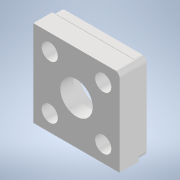
# Autodesk Inventor part: Part8
Saved by Autodesk Inventor 2020.2 (Build 242310000, 310)
## iProperties
Created: 2022-11-14
Part Number: Part8
Material: 一般
Document SubType Name: Modeling
Designer: Administrator
Density: 1 g/cm^3
Appearance: 既定
Author: Administrator
Autodesk Inventor part; units mm, degrees
ref_plane "YZ Plane" through (0, 0, 0) normal (1, 0, 0) x (0, 1, 0)
ref_plane "XZ Plane" through (0, 0, 0) normal (0, 1, 0) x (-1, 0, 0)
ref_plane "XY Plane" through (0, 0, 0) normal (0, 0, 1) x (1, 0, 0)
sketch "スケッチ1" plane through (0, 0, 0) normal (0, 0, 1) x (1, 0, 0)
  circle A0 centre (0.0113, -0.6482) radius 9.5 projected
  circle A1 centre (0.0113, -0.6482) radius 5 projected
  circle A2 centre (0.0113, -0.6482) radius 5 projected
  circle A3 centre (0.0113, -0.6482) radius 14
  circle A4 centre (-9.8882, 9.2513) radius 1.5
  circle A5 centre (9.9108, -10.5477) radius 1.5
  line L0 (0.0113, -0.6482) -> (9.9108, 9.2513)
  line L1 (0.0113, -0.6482) -> (14.0113, -0.6482) construction
  line L2 (0.0113, -0.6482) -> (-9.8882, 9.2513)
  line L3 (0.0113, -0.6482) -> (14.0113, -0.6482) construction
  line L4 (0.0113, -0.6482) -> (-9.8882, -10.5477)
  line L5 (0.0113, -0.6482) -> (14.0113, -0.6482) construction
  line L6 (0.0113, -0.6482) -> (9.9108, -10.5477)
  line L7 (0.0113, -0.6482) -> (14.0113, -0.6482) construction
  circle A6 centre (9.9108, 9.2513) radius 1.5
  circle A7 centre (-9.8882, -10.5477) radius 1.5
  circle A8 centre (-9.8882, 9.2513) radius 3
  circle A9 centre (9.9108, 9.2513) radius 3
  circle A10 centre (9.9108, -10.5477) radius 3
  circle A11 centre (-9.8882, -10.5477) radius 3
  circle A12 centre (0.0113, -0.6482) radius 6
  line L8 (-15.9887, 15.3518) -> (16.0113, 15.3518)
  line L9 (16.0113, 15.3518) -> (16.0113, -16.6482)
  line L10 (16.0113, -16.6482) -> (-15.9887, -16.6482)
  line L11 (-15.9887, -16.6482) -> (-15.9887, 15.3518)
  line L12 (-15.9887, 15.3518) -> (16.0113, -16.6482) construction
  line L13 (16.0113, 15.3518) -> (-15.9887, -16.6482) construction
  point P0 (0, 0)
  dimension "d0" = 28
  dimension "d1" = 3
  dimension "d2" = 3
  dimension "d3" = 45
  dimension "d4" = 135
  dimension "d5" = 135
  dimension "d6" = 45
  dimension "d7" = 3
  dimension "d8" = 3
  dimension "d9" = 6
  dimension "d10" = 6
  dimension "d11" = 6
  dimension "d12" = 6
  dimension "d13" = 12
  dimension "d14" = 32
  dimension "d15" = 32
  constraints: 28 end point, 10 centre point, 8 coincident, 5 horizontal, 4 equal length, 4 point on circle, 2 midpoint, 2 parallel, 1 perpendicular
  measures "d0" diameter of A3
  measures "d1" diameter of A4
  measures "d2" diameter of A5
  measures "d3" angle of L1 L0
  measures "d4" angle of L3 L2
  measures "d5" angle of L4 L5
  measures "d6" angle of L6 L7
  measures "d7" diameter of A6
  measures "d8" diameter of A7
  measures "d9" diameter of A8
  measures "d10" diameter of A9
  measures "d11" diameter of A10
  measures "d12" diameter of A11
  measures "d13" diameter of A12
  measures "d14" distance of L9.end L10.end
  measures "d15" distance of L8.end L9.end
extrude "押し出し1" add sketch "スケッチ1" along normal blind 3 contours A0 L0 A9 A3 A10 L6 | A0 L2 A8 A3 A9 L0 | L6 A10 A3 A11 L4 A0 | A0 L4 A11 A3 A8 L2 | A9 A3 A6 L0 | L0 A6 A3 A9 | A10 A3 A5 L6 | L6 A5 A3 A10 | A8 A3 A4 L2 | L2 A4 A3 A8 | A9 A3 A6 | A11 A3 A7 L4 | L4 A7 A3 A11 | A10 A3 A5 | A8 A3 A4 | A3 A7 A11 | L8 L9 L10 L11
sketch "スケッチ2" plane through (0, 0, 3) normal (0, 0, 1) x (1, 0, 0)
  circle A0 centre (0, -0.75) radius 9.5
  circle A1 centre (0, -0.75) radius 5
  circle A2 centre (0, -0.75) radius 5
  circle A3 centre (0, -0.75) radius 14
  circle A4 centre (-9.8995, 9.1495) radius 1.5
  circle A5 centre (9.8995, -10.6495) radius 1.5
  line L0 (0, -0.75) -> (9.8995, 9.1495)
  line L1 (0, -0.75) -> (14, -0.75) construction
  line L2 (0, -0.75) -> (-9.8995, 9.1495)
  line L3 (0, -0.75) -> (14, -0.75) construction
  line L4 (0, -0.75) -> (-9.8995, -10.6495)
  line L5 (0, -0.75) -> (14, -0.75) construction
  line L6 (0, -0.75) -> (9.8995, -10.6495)
  line L7 (0, -0.75) -> (14, -0.75) construction
  circle A6 centre (9.8995, 9.1495) radius 1.5
  circle A7 centre (-9.8995, -10.6495) radius 1.5
  circle A8 centre (-9.8995, 9.1495) radius 3
  circle A9 centre (9.8995, 9.1495) radius 3
  circle A10 centre (9.8995, -10.6495) radius 3
  circle A11 centre (-9.8995, -10.6495) radius 3
  circle A12 centre (0, -0.75) radius 6
  line L8 (-16, 15.25) -> (16, 15.25)
  line L9 (16, 15.25) -> (16, -16.75)
  line L10 (16, -16.75) -> (-16, -16.75)
  line L11 (-16, -16.75) -> (-16, 15.25)
  line L12 (-16, 15.25) -> (16, -16.75) construction
  line L13 (16, 15.25) -> (-16, -16.75) construction
  point P0 (0, 0)
  point P1 (0, 0)
  dimension "d18" = 28
  dimension "d19" = 3
  dimension "d20" = 3
  dimension "d21" = 45
  dimension "d22" = 135
  dimension "d23" = 135
  dimension "d24" = 45
  dimension "d25" = 3
  dimension "d26" = 3
  dimension "d27" = 6
  dimension "d28" = 6
  dimension "d29" = 6
  dimension "d30" = 6
  dimension "d31" = 12
  dimension "d32" = 32
  dimension "d33" = 32
  constraints: 28 end point, 13 centre point, 8 coincident, 5 horizontal, 4 equal length, 4 point on circle, 2 midpoint, 2 parallel, 1 perpendicular
  measures "d18" diameter of A3
  measures "d19" diameter of A4
  measures "d20" diameter of A5
  measures "d21" angle of L1 L0
  measures "d22" angle of L3 L2
  measures "d23" angle of L4 L5
  measures "d24" angle of L6 L7
  measures "d25" diameter of A6
  measures "d26" diameter of A7
  measures "d27" diameter of A8
  measures "d28" diameter of A9
  measures "d29" diameter of A10
  measures "d30" diameter of A11
  measures "d31" diameter of A12
  measures "d32" distance of L9.end L10.end
  measures "d33" distance of L8.end L9.end
extrude "押し出し2" add sketch "スケッチ2" along normal blind 2 contours A0 L0 A9 A3 A10 L6 | A0 L2 A8 A3 A9 L0 | L6 A10 A3 A11 L4 A0 | A0 L4 A11 A3 A8 L2 | L8 L9 L10 L11
sketch "スケッチ3" plane through (0, 0, 5) normal (0, 0, 1) x (1, 0, 0)
  circle A0 centre (0, -0.75) radius 9.5
  circle A1 centre (0, -0.75) radius 5
  circle A2 centre (0, -0.75) radius 5
  circle A3 centre (0, -0.75) radius 14
  circle A4 centre (-9.8995, 9.1495) radius 1.5
  circle A5 centre (9.8995, -10.6495) radius 1.5
  line L0 (0, -0.75) -> (9.8995, 9.1495)
  line L1 (0, -0.75) -> (14, -0.75) construction
  line L2 (0, -0.75) -> (-9.8995, 9.1495)
  line L3 (0, -0.75) -> (14, -0.75) construction
  line L4 (0, -0.75) -> (-9.8995, -10.6495)
  line L5 (0, -0.75) -> (14, -0.75) construction
  line L6 (0, -0.75) -> (9.8995, -10.6495)
  line L7 (0, -0.75) -> (14, -0.75) construction
  circle A6 centre (9.8995, 9.1495) radius 1.5
  circle A7 centre (-9.8995, -10.6495) radius 1.5
  circle A8 centre (-9.8995, 9.1495) radius 3
  circle A9 centre (9.8995, 9.1495) radius 3
  circle A10 centre (9.8995, -10.6495) radius 3
  circle A11 centre (-9.8995, -10.6495) radius 3
  circle A12 centre (0, -0.75) radius 6
  line L8 (-16, 15.25) -> (16, 15.25)
  line L9 (16, 15.25) -> (16, -16.75)
  line L10 (16, -16.75) -> (-16, -16.75)
  line L11 (-16, -16.75) -> (-16, 15.25)
  line L12 (-16, 15.25) -> (16, -16.75) construction
  line L13 (16, 15.25) -> (-16, -16.75) construction
  point P0 (0, 0)
  point P1 (0, 0)
  point P2 (0, 0)
  dimension "d36" = 28
  dimension "d37" = 3
  dimension "d38" = 3
  dimension "d39" = 45
  dimension "d40" = 135
  dimension "d41" = 135
  dimension "d42" = 45
  dimension "d43" = 3
  dimension "d44" = 3
  dimension "d45" = 6
  dimension "d46" = 6
  dimension "d47" = 6
  dimension "d48" = 6
  dimension "d49" = 12
  dimension "d50" = 32
  dimension "d51" = 32
  constraints: 28 end point, 13 centre point, 8 coincident, 5 horizontal, 4 equal length, 4 point on circle, 2 midpoint, 2 parallel, 1 perpendicular
  measures "d36" diameter of A3
  measures "d37" diameter of A4
  measures "d38" diameter of A5
  measures "d39" angle of L1 L0
  measures "d40" angle of L3 L2
  measures "d41" angle of L4 L5
  measures "d42" angle of L6 L7
  measures "d43" diameter of A6
  measures "d44" diameter of A7
  measures "d45" diameter of A8
  measures "d46" diameter of A9
  measures "d47" diameter of A10
  measures "d48" diameter of A11
  measures "d49" diameter of A12
  measures "d50" distance of L9.end L10.end
  measures "d51" distance of L8.end L9.end
extrude "押し出し3" add sketch "スケッチ3" along normal blind 5 contours A0 L6 A12 L0 | A0 L0 A9 A3 A10 L6 | L0 A12 L2 A0 | A0 L2 A8 A3 A9 L0 | L6 A10 A3 A11 L4 A0 | A0 L4 A12 L6 | L2 A12 L4 A0 | A0 L4 A11 A3 A8 L2 | L8 L9 L10 L11
fillet "フィレット1" radius 2 4 edges at (-15.9887, 15.3518, 1.5) (16.0113, 15.3518, 1.5) (16.0113, -16.6482, 1.5) (-15.9887, -16.6482, 1.5)
